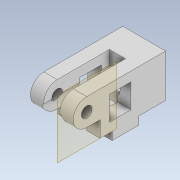
# Autodesk Inventor part: 合页01
Saved by Autodesk Inventor 2022.5 (Build 265521000, 521)
## iProperties
Created: 2024-01-06
Part Number: 合页01
Material: 常规
Document SubType Name: Modeling
Designer: Gagouking
Density: 1 g/cm^3
Appearance: 默认
Author: Gagouking
Autodesk Inventor part; units mm, degrees
ref_plane "YZ Plane" through (0, 0, 0) normal (1, 0, 0) x (0, 1, 0)
ref_plane "XZ Plane" through (0, 0, 0) normal (0, 1, 0) x (-1, 0, 0)
ref_plane "XY Plane" through (0, 0, 0) normal (0, 0, 1) x (1, 0, 0)
sketch "草图1" plane through (0, 0, 0) normal (0, 1, 0) x (-1, 0, 0)
  circle A0 centre (0, 0) radius 1.5
  line L0 (0, 0) -> (-50, 0) construction
  circle A1 centre (-50, 0) radius 1.5
  line L1 (5, -5) -> (-55, -5)
  line L2 (-55, -5) -> (-55, 5)
  line L3 (-55, 5) -> (5, 5)
  line L4 (5, 5) -> (5, -5)
  line L5 (-25, 0) -> (-25, -6.3237) construction
  dimension "d0" = 3
  dimension "d1" = 50
  dimension "d2" = 3
  dimension "d3" = 10
  dimension "d4" = 60
  constraints: 12 end point, 2 centre point, 2 coincident, 2 horizontal, 2 parallel, 1 midpoint, 1 perpendicular, 1 vertical, 2 other
  measures "d0" diameter of A0
  measures "d1" distance of L0.start L0.end
  measures "d2" diameter of A1
  measures "d3" diameter of L1 L0
  measures "d4" diameter of L2 L5
extrude "拉伸1" add sketch "草图1" along normal blind 6
sketch "草图2" plane through (0, 6, 0) normal (0, 1, 0) x (1, 0, 0)
  line L0 (-5, -5) -> (55, -5) projected
  line L1 (55, -5) -> (55, 5) projected
  line L2 (55, 5) -> (-5, 5) projected
  line L3 (-5, 5) -> (-5, -5) projected
  circle A0 centre (50, 0) radius 1.5 projected
  circle A1 centre (0, 0) radius 1.5 projected
  line L4 (55, 5) -> (-5, 5) projected
  line L5 (-5, -5) -> (55, -5) projected
  line L6 (17, 5) -> (22, 5)
  line L7 (22, 5) -> (22, -5)
  line L8 (22, -5) -> (17, -5)
  line L9 (17, -5) -> (17, 5)
  line L10 (28, 5) -> (33, 5)
  line L11 (33, 5) -> (33, -5)
  line L12 (33, -5) -> (28, -5)
  line L13 (28, -5) -> (28, 5)
  line L14 (25, -5) -> (25, 2.8466) construction
  line L15 (17, -5) -> (22, -5)
  line L16 (22, -5) -> (22, -29.5)
  line L17 (22, -29.5) -> (17, -29.5)
  line L18 (17, -29.5) -> (17, -5)
  line L19 (33, -5) -> (28, -5)
  line L20 (28, -5) -> (28, -29.5)
  line L21 (28, -29.5) -> (33, -29.5)
  line L22 (33, -29.5) -> (33, -5)
  point P0 (28, 5)
  point P1 (28, -5)
  point P2 (33, -5)
  point P3 (33, 5)
  point P4 (17, 5)
  point P5 (22, 5)
  point P6 (33, -5)
  dimension "d7" = 5
  dimension "d8" = 6
  dimension "d24" = 24.5
  constraints: 34 end point, 8 parallel, 4 horizontal, 4 perpendicular, 4 point on line, 3 collinear, 1 midpoint, 1 vertical, 2 other
  measures "d7" distance of L7.end L8.end
  measures "d8" diameter of L7 L14
  measures "d24" distance between parallel lines of L0 L21
extrude "拉伸2" add sketch "草图2" along normal blind 10 contours L9 L2 L7 L0 | L0 L16 L17 L18 | L7 L2 L13 L0 | L13 L2 L11 L0 | L0 L22 L21 L20
chamfer "倒角1" distance 2 angle 45 2 edges at (1.5, 6, 0) (51.5, 6, 0)
sketch "草图4" plane through (33, 6, 29.5) normal (1, 0, 0) x (0, 0, -1)
  circle A0 centre (5, 5) radius 2
  line L0 (0, 0) -> (0, 10) projected
  line L1 (0, 5) -> (5, 5)
  point P0 (29.5, -6)
  dimension "d25" = 4
  dimension "d26" = 5
  constraints: 2 end point, 1 centre point, 1 coincident, 1 horizontal, 1 midpoint
  measures "d25" diameter of A0
  measures "d26" distance of L1.start L1.end
extrude "拉伸4" cut sketch "草图4" against normal through all
fillet "圆角7" radius 5 4 edges at (30.5, 16, 29.5) (19.5, 16, 29.5) (19.5, 6, 29.5) (30.5, 6, 29.5)
sketch "草图5" plane through (0, 6, 0) normal (0, -1, 0) x (1, 0, 0)
  line L0 (17, 24.5) -> (22, 24.5) projected
  line L1 (17, 5) -> (17, 24.5) projected
  line L2 (17, 5) -> (22, 5) projected
  line L3 (22, 24.5) -> (22, 5) projected
  line L4 (28, 24.5) -> (33, 24.5) projected
  line L5 (28, 5) -> (28, 24.5) projected
  line L6 (28, 5) -> (33, 5) projected
  line L7 (33, 24.5) -> (33, 5) projected
  line L8 (17, 19.5) -> (33, 19.5)
  line L9 (33, 24.5) -> (33, 5) projected
  line L10 (-5, 5) -> (55, 5) projected
  point P0 (0, 0)
  point P1 (22, 19.5)
  point P2 (28, 19.5)
  dimension "d30" = 14.5
  constraints: 2 end point, 2 point on line, 1 perpendicular
  measures "d30" distance between parallel lines of L10 L8
extrude "拉伸5" add sketch "草图5" along normal blind 6 contours L8 L3 L2 L1 | L8 L7 L6 L5
sketch "草图6" plane through (0, 0, 0) normal (0, -1, 0) x (1, 0, 0)
  line L0 (-5, 5) -> (17, 5) projected
  line L1 (-5, -5) -> (-5, 5) projected
  line L2 (55, -5) -> (-5, -5) projected
  line L3 (55, 5) -> (55, -5) projected
  line L4 (33, 5) -> (55, 5) projected
  line L5 (33, 5) -> (33, 19.5) projected
  line L6 (33, 19.5) -> (28, 19.5) projected
  line L7 (28, 19.5) -> (28, 5) projected
  line L8 (22, 5) -> (28, 5) projected
  line L9 (22, 5) -> (22, 19.5) projected
  line L10 (22, 19.5) -> (17, 19.5) projected
  line L11 (17, 19.5) -> (17, 5) projected
  circle A0 centre (50, 0) radius 1.5 projected
  circle A1 centre (0, 0) radius 1.5 projected
  line L12 (17, 19.5) -> (17, 5) projected
  line L13 (17, 15) -> (33, 15)
  line L14 (33, 5) -> (33, 19.5) projected
  line L15 (17, 5) -> (33, 5)
  point P0 (28, 15)
  point P1 (22, 15)
  dimension "d34" = 10
  constraints: 4 end point, 2 horizontal, 2 point on line
  measures "d34" distance between parallel lines of L8 L13
extrude "拉伸6" add sketch "草图6" along normal blind 3 contours L11 L13 L9 L15 | L7 L13 L5 L15
ref_plane "工作平面1" through (33, 11, 24.5) normal (1, 0, 0) x (0, 0, -1)
sketch "草图7" plane through (33, 11, 24.5) normal (1, 0, 0) x (0, 0, -1)
  circle A0 centre (0, 0) radius 2 projected
  line L0 (8.5, 1.5) -> (16.5, 1.5)
  line L1 (16.5, 1.5) -> (16.5, -7.5)
  line L2 (16.5, -7.5) -> (8.5, -7.5)
  line L3 (8.5, -7.5) -> (8.5, 1.5)
  point P0 (24.5, -11)
  dimension "d43" = 8
  dimension "d44" = 9
  constraints: 8 end point, 2 parallel, 1 horizontal, 1 perpendicular
  measures "d43" distance of L0.start L0.end
  measures "d44" distance of L0.end L1.end
extrude "拉伸7" cut sketch "草图7" against normal through all contours L0 L1 L2 L3
sketch "草图8" plane through (55, 0, -5) normal (0, 0, -1) x (-1, 0, 0)
  line L0 (0, 0) -> (60, 0) projected
  line L1 (60, 0) -> (60, 6) projected
  line L2 (38, 6) -> (60, 6) projected
  line L3 (38, 6) -> (38, 16) projected
  line L4 (22, 16) -> (38, 16) projected
  line L5 (22, 6) -> (22, 16) projected
  line L6 (0, 6) -> (22, 6) projected
  line L7 (0, 0) -> (0, 6) projected
  line L8 (22, 6) -> (22, 16) projected
  line L9 (38, 0) -> (38, -3) projected
  line L10 (22, 16) -> (38, 16)
  line L11 (38, 16) -> (38, 0)
  line L12 (38, 0) -> (22, 0)
  line L13 (22, 0) -> (22, 16)
  circle A0 centre (30, 8) radius 4
  line L14 (30, 8) -> (30, 0) construction
  line L15 (30, 8) -> (22, 8) construction
  line L16 (0, 0) -> (60, 0) projected
  point P0 (55, 0)
  dimension "d50" = 8
  constraints: 12 end point, 2 horizontal, 2 midpoint, 2 parallel, 1 centre point, 1 perpendicular, 1 vertical
  measures "d50" diameter of A0
extrude "拉伸8" cut sketch "草图8" against normal through all contours L7 L6 L13 L0 | L11 L2 L1 L0 | A0
